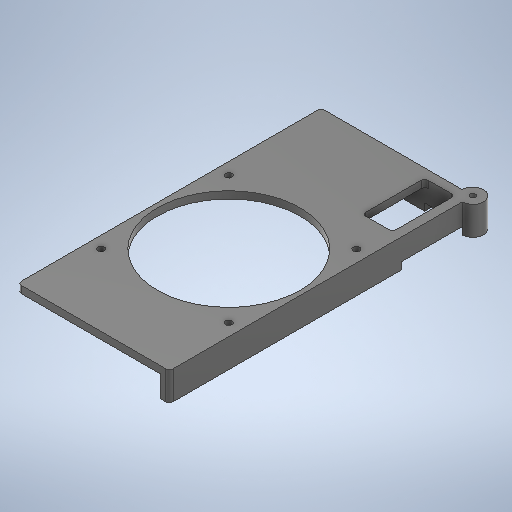
# Autodesk Inventor part: Power Box (24V) Cover
Saved by Autodesk Inventor 2026.2 (Build 302298010, 298A)
## iProperties
Created: 2026-05-26
Part Number: Power Box (24V) Cover
Material: ABS Plastic
Document SubType Name: Modeling
Designer: chanh
Density: 1.06 g/cm^3
Appearance: Smooth - White
Author: chanh
Autodesk Inventor part; units mm, degrees
ref_plane "YZ Plane" through (0, 0, 0) normal (1, 0, 0) x (0, 1, 0)
ref_plane "XZ Plane" through (0, 0, 0) normal (0, 1, 0) x (-1, 0, 0)
ref_plane "XY Plane" through (0, 0, 0) normal (0, 0, 1) x (1, 0, 0)
sketch "Sketch1" plane through (0, 0, 0) normal (0, 1, 0) x (-1, 0, 0)
  line L0 (42.5, 85) -> (-42.5, 85)
  line L1 (-42.5, 85) -> (-42.5, -85)
  line L2 (-42.5, -85) -> (42.5, -85)
  line L3 (42.5, -85) -> (42.5, 85)
  line L4 (42.5, 85) -> (-42.5, -85) construction
  line L5 (-42.5, 85) -> (42.5, -85) construction
  circle A0 centre (-42.5, -85) radius 6
  point P0 (0, 0)
  point P1 (-42.5, -79)
  point P2 (-36.5, -85)
  dimension "d0" = 85
  dimension "d1" = 170
  dimension "d2" = 12
  constraints: 12 end point, 2 midpoint, 2 parallel, 1 centre point, 1 coincident, 1 horizontal, 1 perpendicular
  measures "d0" distance of L2.end L1.end
  measures "d1" distance of L0.end L1.end
  measures "d2" diameter of A0
extrude "Extrusion1" add sketch "Sketch1" along normal blind 4
sketch "Sketch2" plane through (0, 0, 0) normal (0, -1, 0) x (1, 0, 0)
  line L0 (42.5, 85) -> (42.5, -79) projected
  line L1 (-42.5, 85) -> (42.5, 85) projected
  line L2 (-42.5, -85) -> (-42.5, 85) projected
  line L3 (36.5, -85) -> (-42.5, -85) projected
  arc A0 (36.5, -85) -> (42.5, -79) centre (42.5, -85) ccw projected
  line L4 (37.5, 85) -> (37.5, -80)
  line L5 (37.5, -80) -> (-42.5, -80)
  point P0 (0, 0)
  dimension "d5" = 5
  dimension "d6" = 5
  constraints: 4 end point, 2 point on line, 1 perpendicular, 1 vertical
  measures "d5" distance between parallel lines of L3 L5
  measures "d6" distance between parallel lines of L0 L4
extrude "Extrusion2" add sketch "Sketch2" along normal blind 12 contours L0 A0 L3 L2 L5 L4 L1
sketch "Sketch3" plane through (0, 4, 0) normal (0, 1, 0) x (1, 0, 0)
  arc A0 (42.5, 79) -> (36.5, 85) centre (42.5, 85) ccw projected
  arc A1 (42.5, 79) -> (36.5, 85) centre (42.5, 85) ccw projected
  point P0 (0, 0)
hole "Hole1" at (42.5, 4, -85) direction (0, -1, 0) diameter 3.2 end through all
sketch "Sketch4" plane through (0, 4, 0) normal (0, 1, 0) x (1, 0, 0)
  line L0 (35.75, -45) -> (-35.75, -45) construction
  line L1 (-35.75, -45) -> (-35.75, 26.5) construction
  line L2 (-35.75, 26.5) -> (35.75, 26.5) construction
  line L3 (35.75, 26.5) -> (35.75, -45) construction
  line L4 (35.75, -45) -> (-35.75, 26.5) construction
  line L5 (-35.75, -45) -> (35.75, 26.5) construction
  circle A0 centre (42.5, 85) radius 1.6 projected
  line L6 (42.5, -85) -> (42.5, 79) projected
  arc A1 (42.5, 79) -> (36.5, 85) centre (42.5, 85) ccw projected
  line L7 (36.5, 85) -> (-42.5, 85) projected
  line L8 (-42.5, 85) -> (-42.5, -85) projected
  line L9 (-42.5, -85) -> (42.5, -85) projected
  point P0 (0, 0)
  point P1 (0, -9.25)
  dimension "d16" = 71.5
  dimension "d17" = 40
  constraints: 12 end point, 4 coincident, 2 midpoint, 2 parallel, 2 perpendicular, 1 horizontal, 1 vertical alignment
  measures "d16" distance of L0.end L1.end
  measures "d17" distance between parallel lines of L9 L0
hole "Hole2" at (-35.75, 4, 45) at (-35.75, 4, -26.5) at (35.75, 4, 45) at (35.75, 4, -26.5) direction (0, -1, 0) diameter 3.7 depth 4 tip angle 118
sketch "Sketch5" plane through (0, 4, 0) normal (0, 1, 0) x (1, 0, 0)
  circle A0 centre (0, -9.25) radius 40
  point P0 (0, 0)
  dimension "d25" = 80
  constraints: 1 centre point, 1 coincident
  measures "d25" diameter of A0
extrude "Extrusion3" cut sketch "Sketch5" against normal up to surface (4 mm away)
sketch "Sketch6" plane through (0, -12, 0) normal (0, -1, 0) x (1, 0, 0)
  circle A0 centre (42.5, -85) radius 1.6 projected
  line L0 (42.5, 85) -> (37.5, 85) projected
  line L1 (37.5, 85) -> (37.5, -80) projected
  line L2 (37.5, -80) -> (-42.5, -80) projected
  line L3 (-42.5, -80) -> (-42.5, -85) projected
  line L4 (-42.5, -85) -> (36.5, -85) projected
  arc A1 (36.5, -85) -> (42.5, -79) centre (42.5, -85) ccw projected
  line L5 (42.5, -79) -> (42.5, 85) projected
  line L6 (42.5, -45) -> (37.5, -45)
  line L7 (20.5, -85) -> (20.5, -80)
  line L8 (42.5, -85) -> (36.5, -85)
  line L9 (42.5, -85) -> (42.5, -79)
  point P0 (0, 0)
  point P1 (42.5, -83.4)
  point P2 (40.9, -85)
  dimension "d28" = 22
  dimension "d29" = 40
  constraints: 8 end point, 4 point on line, 2 perpendicular, 1 collinear, 1 horizontal
  measures "d28" distance between parallel lines of L7 L5
  measures "d29" distance between parallel lines of L6 L4
extrude "Extrusion4" cut sketch "Sketch6" against normal blind 4 contours A0 L8 L4 L7 L2 L1 L6 L5 L9
sketch "Sketch7" plane through (0, -8, 0) normal (0, -1, 0) x (1, 0, 0)
  line L0 (42.5, -45) -> (42.5, -79) projected
  line L1 (37.5, -45) -> (42.5, -45) projected
  line L2 (37.5, -80) -> (37.5, -45) projected
  line L3 (20.5, -80) -> (37.5, -80) projected
  line L4 (20.5, -85) -> (20.5, -80) projected
  line L5 (36.5, -85) -> (20.5, -85) projected
  line L6 (40.9, -85) -> (36.5, -85) projected
  arc A0 (42.5, -83.4) -> (40.9, -85) centre (42.5, -85) ccw projected
  line L7 (42.5, -79) -> (42.5, -83.4) projected
  line L8 (37.5, -80) -> (20.5, -80)
  line L9 (20.5, -80) -> (20.5, -45)
  line L10 (20.5, -45) -> (37.5, -45)
  line L11 (37.5, -45) -> (37.5, -80)
  line L12 (37.5, -45) -> (42.5, -45) projected
  line L13 (20.5, -85) -> (20.5, -80) projected
  point P0 (0, 0)
  constraints: 8 end point, 2 collinear, 2 parallel, 1 horizontal, 1 perpendicular
extrude "Extrusion5" cut sketch "Sketch7" against normal through all contours L2 L3 L9 L10
fillet "Fillet1" radius 2 7 edges at (37.5, 2, -45) (20.5, 2, -45) (37.5, -2, -80) (20.5, 2, -80) (-42.5, -4, -85) (-42.5, 2, 85) (42.5, -4, 85)
equation "\"d6\" = d5"
body "Solid1"
